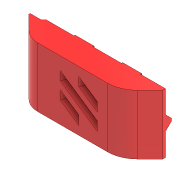
# Autodesk Inventor part: Cover
Saved by Autodesk Inventor 2021 (Build 250183000, 183)
## iProperties
Created: 2021-08-30
Part Number: Cover
Material: Generisch
Document SubType Name: Modeling
Designer: Rama
Density: 1 g/cm^3
Appearance: Hellrot
Author: Rama
Autodesk Inventor part; units mm, degrees
ref_plane "YZ Plane" through (0, 0, 0) normal (1, 0, 0) x (0, 1, 0)
ref_plane "XZ Plane" through (0, 0, 0) normal (0, 1, 0) x (-1, 0, 0)
ref_plane "XY Plane" through (0, 0, 0) normal (0, 0, 1) x (1, 0, 0)
sketch "Skizze1" plane through (0, 0, 0) normal (0, 0, 1) x (1, 0, 0)
  line L0 (-4.2865, -7.5) -> (-4.2865, -10) projected
  line L1 (5.2135, -10) -> (-4.2865, -10) projected
  line L2 (5.2135, -10) -> (5.2135, -7.5) projected
  arc A0 (11.7135, -7.5) -> (5.2135, -7.5) centre (8.4635, -7.5) ccw projected
  line L3 (11.7135, -7.5) -> (11.7135, -10) projected
  line L4 (20, -10) -> (11.7135, -10) projected
  line L5 (20, 10) -> (20, -10) projected
  line L6 (11.7135, 10) -> (20, 10) projected
  line L7 (11.7135, 10) -> (11.7135, 7.5) projected
  arc A1 (5.2135, 7.5) -> (11.7135, 7.5) centre (8.4635, 7.5) ccw projected
  line L8 (5.2135, 7.5) -> (5.2135, 10) projected
  line L9 (-4.2865, 10) -> (5.2135, 10) projected
  line L10 (-4.2865, 10) -> (-4.2865, 7.5) projected
  arc A2 (-10.7865, 7.5) -> (-4.2865, 7.5) centre (-7.5365, 7.5) ccw projected
  line L11 (-10.7865, 7.5) -> (-10.7865, 10) projected
  line L12 (-20, 10) -> (-10.7865, 10) projected
  line L13 (-20, -10) -> (-20, 10) projected
  line L14 (-10.7865, -10) -> (-20, -10) projected
  line L15 (-10.7865, -10) -> (-10.7865, -7.5) projected
  arc A3 (-4.2865, -7.5) -> (-10.7865, -7.5) centre (-7.5365, -7.5) ccw projected
  circle A4 centre (-7.5365, 7.5) radius 3.2
  circle A5 centre (8.4635, 7.5) radius 3.2
  circle A6 centre (8.4635, -7.5) radius 3.2
  circle A7 centre (-7.5365, -7.5) radius 3.2
  line L16 (-10.7365, 7.5) -> (-4.3365, 7.5)
  line L17 (-4.3365, 7.5) -> (-4.3365, 12.5)
  line L18 (-4.3365, 12.5) -> (-10.7365, 12.5)
  line L19 (-10.7365, 12.5) -> (-10.7365, 7.5)
  line L20 (5.2635, 7.5) -> (11.6635, 7.5)
  line L21 (11.6635, 7.5) -> (11.6635, 12.5)
  line L22 (11.6635, 12.5) -> (5.2635, 12.5)
  line L23 (5.2635, 12.5) -> (5.2635, 7.5)
  line L24 (-10.7365, -7.5) -> (-4.3365, -7.5)
  line L25 (-4.3365, -7.5) -> (-4.3365, -12.5)
  line L26 (-4.3365, -12.5) -> (-10.7365, -12.5)
  line L27 (-10.7365, -12.5) -> (-10.7365, -7.5)
  line L28 (5.2635, -7.5) -> (11.6635, -7.5)
  line L29 (11.6635, -7.5) -> (11.6635, -12.5)
  line L30 (11.6635, -12.5) -> (5.2635, -12.5)
  line L31 (5.2635, -12.5) -> (5.2635, -7.5)
  line L32 (20, 10) -> (-19.9, 10)
  line L33 (-19.9, 10) -> (-19.9, -10)
  line L34 (-19.9, -10) -> (20, -10)
  line L35 (20, -10) -> (20, 10)
  circle A8 centre (-3.95, 0) radius 2 projected
  point P0 (0, 0)
  point P1 (-4.3365, -7.5)
  point P2 (-10.7365, -10)
  point P3 (-4.3365, -10)
  point P4 (11.6635, -7.5)
  point P5 (5.2635, -10)
  point P6 (11.6635, -10)
  point P7 (11.6635, 7.5)
  point P8 (11.6635, 10)
  point P9 (5.2635, 10)
  point P10 (-10.7365, 10)
  point P11 (-4.3365, 7.5)
  point P12 (-4.3365, 10)
  dimension "d1" = 6.4
  dimension "d2" = 6.4
  dimension "d3" = 6.4
  dimension "d4" = 6.4
  dimension "d0" = 3.25
  dimension "d5" = 6.4
  dimension "d6" = 5
  dimension "d7" = 5
  dimension "d8" = 6.4
  dimension "d9" = 6.4
  dimension "d10" = 6.4
  dimension "d11" = 5
  dimension "d12" = 5
  dimension "d13" = 0.1
  constraints: 40 end point, 10 parallel, 5 horizontal, 5 perpendicular, 4 coincident, 1 point on line, 12 other
  measures "d0" radius of A2
  measures "d5" distance of L17.end L18.end
  measures "d6" distance of L18.end L16.start
  measures "d7" distance of L22.end L20.start
  measures "d8" distance of L21.end L22.end
  measures "d9" distance of L25.end L26.end
  measures "d10" distance of L29.end L30.end
  measures "d11" distance of L30.end L28.start
  measures "d12" distance of L26.end L24.start
  measures "d13" distance between parallel lines of L13 L33
extrude "Extrusion1" add sketch "Skizze1" against normal blind 0.4 contours L34 A7 L25 | L31 A6 L34 | L24 A7 | A7 L34 L24 | L27 A7 L34 | L28 A6 L34 | A6 L28 | L29 L34 A6 | L32 A4 L19 | L16 A4 | A4 L32 L16 | A4 L32 L17 | L21 A5 L32 | L20 A5 L32 | A5 L20 | L32 A5 L23
ref_plane "Arbeitsebene1" through (0, 0, 0) normal (0, 0, 1) x (1, 0, 0)
sketch "Skizze2" plane through (0, 0, 0) normal (0, 0, 1) x (1, 0, 0)
  line L0 (-4.2865, -7.5) -> (-4.2865, -10) projected
  line L1 (5.2135, -10) -> (-4.2865, -10) projected
  line L2 (5.2135, -10) -> (5.2135, -7.5) projected
  arc A0 (11.7135, -7.5) -> (5.2135, -7.5) centre (8.4635, -7.5) ccw projected
  line L3 (11.7135, -7.5) -> (11.7135, -10) projected
  line L4 (20, -10) -> (11.7135, -10) projected
  line L5 (20, 10) -> (20, -10) projected
  line L6 (11.7135, 10) -> (20, 10) projected
  line L7 (11.7135, 10) -> (11.7135, 7.5) projected
  arc A1 (5.2135, 7.5) -> (11.7135, 7.5) centre (8.4635, 7.5) ccw projected
  line L8 (5.2135, 7.5) -> (5.2135, 10) projected
  line L9 (-4.2865, 10) -> (5.2135, 10) projected
  line L10 (-4.2865, 10) -> (-4.2865, 7.5) projected
  arc A2 (-10.7865, 7.5) -> (-4.2865, 7.5) centre (-7.5365, 7.5) ccw projected
  line L11 (-10.7865, 7.5) -> (-10.7865, 10) projected
  line L12 (-20, 10) -> (-10.7865, 10) projected
  line L13 (-20, -10) -> (-20, 10) projected
  line L14 (-10.7865, -10) -> (-20, -10) projected
  line L15 (-10.7865, -10) -> (-10.7865, -7.5) projected
  arc A3 (-4.2865, -7.5) -> (-10.7865, -7.5) centre (-7.5365, -7.5) ccw projected
  line L16 (20, 10) -> (-19.9, 10)
  line L17 (-19.9, 10) -> (-19.9, -10)
  line L18 (-19.9, -10) -> (20, -10)
  line L19 (20, -10) -> (20, 10)
  circle A4 centre (-3.95, 0) radius 2 projected
  point P0 (0, 0)
  dimension "d16" = 0.1
  constraints: 8 end point, 2 parallel, 1 horizontal, 1 perpendicular, 1 point on line
  measures "d16" distance between parallel lines of L13 L17
extrude "Extrusion2" add sketch "Skizze2" along normal blind 7.9 contours A3 L15 L14 L17 L12 L11 A2 L10 L9 L8 A1 L7 L6 L5 L4 L3 A0 L2 L1 L0 | L0 L18 L15 A3 | L2 A0 L3 L18 | L16 L10 A2 L11 | L7 A1 L8 L16 | A4
chamfer "Fase1" distance 7 angle 45 1 edges at (20, 0, 7.9)
sketch "Skizze3" plane through (5.2635, 10, -0.4) normal (0, 1, 0) x (1, 0, 0)
  line L0 (-31.7635, -2.7) -> (-34.2635, -0.2) projected
  line L1 (-30.2635, -1.2) -> (-26.0635, -1.2) projected
  line L2 (-25.2635, -0.4) -> (-26.0635, -1.2) projected
  line L3 (-34.2635, -0.2) -> (-26.1635, -8.3)
  line L4 (-34.2635, -0.2) -> (-22.8084, -0.2) construction
  line L5 (-25.1635, -8.3) -> (7.7365, -8.3) projected
  line L6 (-22, -8.3) -> (-26.1635, -8.3)
  line L7 (-25.1635, -0.4) -> (-25.1635, -8.3) projected
  line L8 (-33.2135, -1.25) -> (-26.0428, -1.25)
  line L9 (-26.0428, -1.25) -> (-25.1928, -0.4)
  line L10 (-26.0428, -1.25) -> (-24.8407, -1.25) construction
  line L11 (-25.1635, -0.4) -> (-25.1928, -0.4)
  line L12 (-32.8135, -1.65) -> (-32.8135, -1.25)
  point P0 (-5.2635, -0.4)
  dimension "d22" = 45
  dimension "d23" = 0.05
  dimension "d24" = 45
  dimension "d25" = 0.05
  dimension "d26" = 0.4
  constraints: 16 end point, 10 point on line, 3 horizontal, 2 equal length, 1 collinear, 1 parallel, 1 vertical
  measures "d22" angle of L3 L4
  measures "d23" distance between parallel lines of L1 L8
  measures "d24" angle of L10 L9
  measures "d25" distance from line of L2.start L9
  measures "d26" distance of L12.start L12.end
extrude "Extrusion3" add sketch "Skizze3" against normal up to surface (20 mm away) contours L0 L12 L8 L9 L11 L7 L6 L3
move faces "Verschieben1" translate (0, 0, 0.2) faces at (-9.6, 3.3333, 7.9)
fillet "Rundung1" radius 10 2 edges at (-20.7, 0, 8.1) (12.8, 0, 8.1)
sketch "Skizze4" plane through (-16.5579, 10, 8.1) normal (0, 0, 1) x (1, 0, 0)
  line L0 (25.2157, 0) -> (25.2157, -20) projected
  line L1 (25.2157, 0) -> (0, 0) projected
  line L2 (0, -20) -> (0, 0) projected
  line L3 (0, -20) -> (25.2157, -20) projected
  line L4 (15.6079, -17.1087) -> (9.4084, -12.8877)
  line L5 (15.6079, -17.1087) -> (23.1079, -17.1087) construction
  line L6 (9.4084, -12.8877) -> (9.4084, -9.8877)
  line L7 (9.4084, -9.8877) -> (15.6079, -14.1087)
  line L8 (15.6079, -14.1087) -> (15.6079, -17.1087)
  line L9 (21.8073, -15.721) -> (9.4084, -7.279)
  line L10 (9.4084, -7.279) -> (9.4084, -4.279)
  line L11 (9.4084, -4.279) -> (21.8073, -12.721)
  line L12 (21.8073, -15.721) -> (21.8073, -12.721)
  line L13 (21.8073, -10.1123) -> (15.6079, -5.8913)
  line L14 (15.6079, -5.8913) -> (15.6079, -2.8913)
  line L15 (15.6079, -2.8913) -> (21.8073, -7.1123)
  line L16 (21.8073, -7.1123) -> (21.8073, -10.1123)
  line L17 (9.4084, -17.1087) -> (21.8073, -17.1087)
  line L18 (21.8073, -17.1087) -> (21.8073, -2.8913)
  line L19 (21.8073, -2.8913) -> (9.4084, -2.8913)
  line L20 (9.4084, -2.8913) -> (9.4084, -17.1087)
  line L21 (0, -20) -> (0, 0) projected
  line L22 (0, -20) -> (12.6079, -20)
  line L23 (12.6079, -20) -> (12.6079, -10)
  line L24 (12.6079, -10) -> (0, -10)
  line L25 (0, -10) -> (0, -20)
  circle A0 centre (12.6079, -10) radius 2.8
  point P0 (16.5579, -10)
  dimension "d97" = 145.75
  dimension "d99" = 3
  dimension "d102" = 2.6087
  dimension "d103" = 7.5
  dimension "d104" = 15
  dimension "d106" = 0
  dimension "d110" = 3
  dimension "d111" = 15
  dimension "d113" = 3
  dimension "d114" = 7.5
  dimension "d118" = 0
  dimension "d119" = 2.6087
  dimension "d124" = 12.3988
  dimension "d125" = 14.2174
  dimension "d126" = 25.2157
  dimension "d127" = 20
  dimension "d128" = 3.4084
  dimension "d129" = 2.8913
  dimension "d146" = 20
  dimension "d147" = 10
  dimension "d148" = 12.6079
  dimension "d149" = 5.6
  constraints: 42 end point, 11 parallel, 3 horizontal, 3 vertical, 2 midpoint, 2 perpendicular, 2 point on line, 1 centre point, 1 coincident, 1 equal length
  measures "d97" angle of L5 L4
  measures "d99" distance of L4.end L6.end
  measures "d102" distance of L9.end L6.end
  measures "d103" distance of L4.start L4.end
  measures "d104" distance of L9.start L9.end
  measures "d106" distance from line of L9.end L6
  measures "d110" distance of L9.end L10.end
  measures "d111" distance of L10.end L11.end
  measures "d113" distance of L14.start L14.end
  measures "d114" distance of L13.start L14.start
  measures "d118" distance from line of L13.start L12
  measures "d119" distance of L13.start L11.end
  measures "d124" distance of L17.start L17.end
  measures "d125" distance of L19.end L17.start
  measures "d126" distance of L2.start L0.end
  measures "d127" distance of L0.start L0.end
  measures "d128" distance between parallel lines of L0 L18
  measures "d129" distance between parallel lines of L1 L19
  measures "d146" distance of L2.start L1.end
  measures "d147" distance of L22.end L23.end
  measures "d148" distance of L23.end L24.end
  measures "d149" diameter of A0
extrude "Extrusion4" cut sketch "Skizze4" against normal blind 1 contours L24 L7 A0 L23 L4 L6 | L6 L7 L24 | L4 L23 A0 L7 L8 | A0 L7 L23 | L23 L7 A0 | L10 L11 L12 L9 A0 | A0 L9 | L13 L14 L15 L16
chamfer "Fase3" distance 1 angle 45 12 edges at (5.2494, 1.3877, 7.1) (2.1497, 1.9982, 7.1) (-0.95, 5.6087, 7.1) (2.1497, 4.9982, 7.1) (5.2494, -4.221, 7.1) (-0.95, -1.5, 7.1) (-0.95, 1.5, 7.1) (-7.1494, 4.221, 7.1) (-4.0497, -1.9982, 7.1) (-0.95, -5.6087, 7.1) (-4.0497, -4.9982, 7.1) (-7.1494, -1.3877, 7.1)
delete faces "Fläche löschen1" heal yes whole lump no faces at (-19.7723, 3.3333, 7.5693) (-26.243, -3.3333, 2.557)
sketch "Skizze8" plane through (-4.3365, 10, 0) normal (0, 1, 0) x (1, 0, 0)
  line L0 (-20.6635, -0.8) -> (-22.2535, 0.7899) projected
  line L1 (-23.5398, 2.0762) -> (-12.3017, -9.1618)
  line L2 (12.9943, -8.1) -> (-23.2135, -8.1) projected
  line L3 (-23.2135, -0.85) -> (-23.2135, -8.1) projected
  line L4 (-16.4428, -0.85) -> (-23.2135, -0.85) projected
  line L5 (-20.2135, -1.25) -> (-20.2135, -0.85)
  point P0 (4.3365, 0)
  point P1 (-7.9648, -8.1)
  point P2 (-13.3635, -8.1)
  dimension "d167" = 0
  dimension "d168" = 0.4
  constraints: 4 end point, 2 point on line, 1 collinear, 1 vertical
  measures "d167" distance between parallel lines of L0 L1
  measures "d168" distance of L5.start L5.end
extrude "Extrusion7" cut sketch "Skizze8" against normal through all
fillet "Rundung4" radius 7 1 edges at (-17.7, 0, 8.1)
sketch "Skizze9" plane through (20, -10, 0) normal (1, 0, 0) x (0, 0, -1)
  line L0 (2, 9.5) -> (0, 7.5)
  line L1 (2, 10.5) -> (2, 9.5)
  line L2 (0, 12.5) -> (2, 10.5)
  line L3 (0, 0) -> (0, 20)
  line L4 (0, 12.4293) -> (1.99, 10.4393)
  line L5 (1.99, 10.4393) -> (1.99, 9.5607)
  line L6 (-0.9, 0) -> (-0.9, 20)
  line L7 (1.99, 9.5607) -> (0, 7.5707)
  point P0 (0, 10)
  dimension "d172" = 0.01
  dimension "d173" = 0.05
  dimension "d175" = 0.05
  constraints: 16 end point, 2 point on line
  measures "d172" distance between parallel lines of L1 L5
  measures "d173" distance between parallel lines of L2 L4
  measures "d175" distance between parallel lines of L0 L7
extrude "Extrusion8" add sketch "Skizze9" against normal blind 4.95 contours L3 L4 L5 L7
chamfer "Fase5" distance 1.99 angle 45 1 edges at (15.05, 0, 0)
sketch "Skizze10" plane through (0, 0, -0.4) normal (0, 0, -1) x (-1, 0, 0)
  arc A0 (-11.6635, 7.5) -> (-5.2635, 7.5) centre (-8.4635, 7.5) ccw projected
  arc A1 (-5.2635, -7.5) -> (-11.6635, -7.5) centre (-8.4635, -7.5) ccw projected
  arc A2 (10.7365, -7.5) -> (4.3365, -7.5) centre (7.5365, -7.5) ccw projected
  arc A3 (4.3365, 7.5) -> (10.7365, 7.5) centre (7.5365, 7.5) ccw projected
  line L0 (-8.4635, -6) -> (7.5365, -6)
  line L1 (7.5365, -6) -> (7.5365, 6)
  line L2 (7.5365, 6) -> (-8.4635, 6)
  line L3 (-8.4635, 6) -> (-8.4635, -6)
  line L4 (-8.4635, -6) -> (7.5365, 6) construction
  line L5 (7.5365, -6) -> (-8.4635, 6) construction
  circle A4 centre (-8.4635, 6) radius 3.01
  circle A5 centre (7.5365, 6) radius 3.01
  circle A6 centre (7.5365, -6) radius 3.01
  circle A7 centre (-8.4635, -6) radius 3.01
  line L6 (-5.2635, 10) -> (4.3365, 10) projected
  line L7 (4.3365, -10) -> (-5.2635, -10) projected
  point P0 (-0.4635, 0)
  dimension "d181" = 16
  dimension "d182" = 12
  dimension "d183" = 6.02
  dimension "d184" = 6.02
  dimension "d185" = 6.02
  dimension "d186" = 6.02
  dimension "d187" = 16
  dimension "d188" = 15
  dimension "d189" = 0
  dimension "d190" = 4
  dimension "d191" = 20
  constraints: 12 end point, 4 centre point, 4 coincident, 2 midpoint, 2 parallel, 1 horizontal, 1 perpendicular
  measures "d181" distance of L2.end L1.end
  measures "d182" distance of L1.end L0.end
  measures "d183" diameter of A4
  measures "d184" diameter of A7
  measures "d185" diameter of A5
  measures "d186" diameter of A6
  measures "d187" distance of A2.centre A1.centre
  measures "d188" distance of A3.centre A2.centre
  measures "d189" horizontal distance of A0.centre L2.end
  measures "d190" distance between parallel lines of L6 L2
  measures "d191" distance between parallel lines of L7 L6
extrude "Extrusion9" cut sketch "Skizze10" against normal blind 3.2 contours A4 A0 L2 L3 | A0 L3 A4 | L3 L2 A0 | A0 L2 A4 L3 | A4 L2 A0 | A7 L0 A1 L3 | L3 A1 A7 | A5 A3 L2 | L2 A3 L1 A5 | L3 L0 A1 A7 | A1 L0 L3 | A7 A1 L0 | L2 L1 A3 | A3 A5 L1 L2 | L1 A3 A5 | A6 L1 A2 L0 | L0 A2 A6 | A6 A2 L1 | L0 L1 A2 A6 | A2 L1 L0
fillet "Rundung5" radius 0.4 8 edges at (11.4523, 6.3567, -0.2) (5.4747, 6.3567, -0.2) (5.4747, -6.3567, -0.2) (11.4523, -6.3567, -0.2) (-4.5477, -6.3567, -0.2) (-10.5253, -6.3567, -0.2) (-10.5253, 6.3567, -0.2) (-4.5477, 6.3567, -0.2)
sketch "Skizze11" plane through (20, -10, 0.9) normal (1, 0, 0) x (0, 0, -1)
  line L0 (1.3, 17.9463) -> (1.3, 17.5463) projected
  line L1 (0.9, 17.5463) -> (1.3, 17.5463) projected
  line L2 (1.3, 2.4537) -> (0.9, 2.4537) projected
  line L3 (1.3, 2.4537) -> (1.3, 2.0537) projected
  line L4 (0.9, 17.9463) -> (0.9, 17.5463) projected
  line L5 (1.3, 20) -> (1.3, 17.9463) projected
  line L6 (0.9, 17.5463) -> (1.3, 17.9463)
  line L7 (0.9, 17.5463) -> (1.4657, 17.5463) construction
  line L8 (1.3, 2.0537) -> (1.3, 0) projected
  line L9 (0.9, 2.4537) -> (1.3, 2.0537)
  line L10 (0.9, 2.4537) -> (1.4657, 2.4537) construction
  point P0 (0.9, 10)
  point P1 (1.3, 17.718)
  point P2 (1.3, 2.282)
  point P3 (0.9, 17.718)
  dimension "d195" = 45
  dimension "d196" = 45
  constraints: 8 end point, 2 equal length, 2 horizontal
  measures "d195" angle of L7 L6
  measures "d196" angle of L9 L10
extrude "Extrusion10" cut sketch "Skizze11" against normal through all
equation "\"d2\" = d1"
equation "\"d3\" = d1"
equation "\"d4\" = d1"
equation "\"d5\" = d1"
equation "\"d7\" = d6"
equation "\"d8\" = d1"
equation "\"d9\" = d1"
equation "\"d10\" = d9"
equation "\"d11\" = d6"
equation "\"d12\" = d6"
